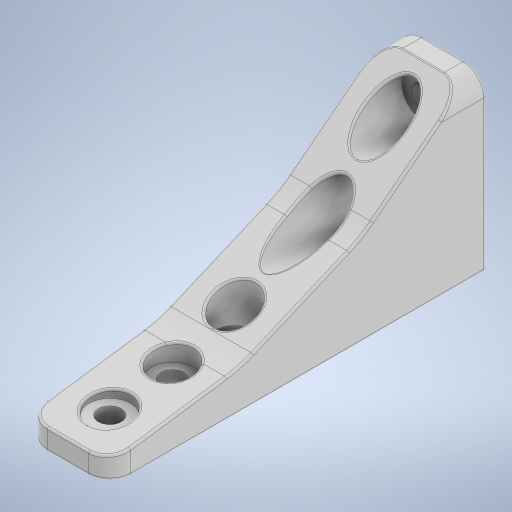
# Autodesk Inventor part: BraketBack
Saved by Autodesk Inventor 2024 (Build 280153000, 153)
## iProperties
Created: 2023-12-26
Part Number: BraketBack
Material: Generisch
Document SubType Name: Modeling
Designer: denni
Density: 1 g/cm^3
Appearance: Vorgabe
Author: denni
Autodesk Inventor part; units mm, degrees
ref_plane "YZ Plane" through (0, 0, 0) normal (1, 0, 0) x (0, 1, 0)
ref_plane "XZ Plane" through (0, 0, 0) normal (0, 1, 0) x (-1, 0, 0)
ref_plane "XY Plane" through (0, 0, 0) normal (0, 0, 1) x (1, 0, 0)
sketch "Skizze1" plane through (0, 0, 0) normal (1, 0, 0) x (0, 1, 0)
  line L0 (0, 90) -> (0, 0)
  line L1 (0, 0) -> (41, 0)
  line L2 (41, 0) -> (41, 5)
  line L3 (0, 90) -> (5, 90)
  line L4 (5, 90) -> (9.3569, 58.8179)
  line L5 (9.3569, 58.8179) -> (21.6358, 29.826)
  line L6 (21.6358, 29.826) -> (41, 5)
  dimension "d0" = 90
  dimension "d1" = 41
  dimension "d2" = 5
  dimension "d3" = 165
  dimension "d4" = 165
  constraints: 14 end point, 3 equal length, 2 vertical, 1 horizontal, 1 perpendicular
  measures "d0" distance of L0.start L0.end
  measures "d1" distance of L0.end L1.end
  measures "d2" distance of L1.end L2.end
  measures "d3" angle of L5 L6
  measures "d4" angle of L4 L5
extrude "Extrusion1" add sketch "Skizze1" along normal blind 20
fillet "Rundung1" radius 25 2 edges at (10, 9.3569, 58.8179) (10, 21.6358, 29.826)
sketch "Skizze4" plane through (0, 41, 5) normal (0, 1, 0) x (1, 0, 0)
  line L0 (0, -85) -> (20, -85) construction
  line L1 (0, -57.0776) -> (0, -85) construction
  point P0 (0, 5)
  point P1 (10, -75)
  point P2 (10, -60)
  point P3 (10, -45)
  dimension "d10" = 10
  dimension "d11" = 15
  dimension "d12" = 15
  dimension "d13" = 10
  dimension "d14" = 10
  dimension "d15" = 10
  measures "d10" distance from line of L0 point (10, -75)
  measures "d11" distance of point (10, -60) point (10, -75)
  measures "d12" distance of point (10, -45) point (10, -60)
  measures "d13" distance from line of L1 point (10, -75)
  measures "d14" distance from line of L1 point (10, -60)
  measures "d15" distance from line of L1 point (10, -45)
hole "Bohrung1" at (10, 41, 80) at (10, 41, 65) at (10, 41, 50) direction (0, -1, 0) diameter 5.5 end through all counterbore diameter 10 counterbore depth 36 clearance for "Inbusschraube ISO 4762" size "M5" standard "ISO"
sketch "Skizze6" plane through (0, 0, 90) normal (0, 0, 1) x (1, 0, 0)
  line L0 (20, 41) -> (20, 23.6601) projected
  line L1 (0, 41) -> (20, 41) projected
  point P0 (0, 0)
  point P1 (10, 33.5)
  point P2 (10, 21)
  dimension "d23" = 10
  dimension "d24" = 10
  dimension "d25" = 7.5
  dimension "d26" = 12.5
  measures "d23" distance from line of L0 point (10, 33.5)
  measures "d24" distance from line of L0 point (10, 21)
  measures "d25" distance from line of L1 point (10, 33.5)
  measures "d26" distance of point (10, 33.5) point (10, 21)
hole "Bohrung2" at (10, 33.5, 90) at (10, 21, 90) direction (0, 0, -1) diameter 5.5 end through all counterbore diameter 10 counterbore depth 85 clearance for "Inbusschraube ISO 4762" size "M5" standard "ISO"
fillet "Rundung2" radius 5 4 edges at (0, 2.5, 90) (20, 2.5, 90) (0, 41, 2.5) (20, 41, 2.5)
fillet "Rundung3" radius 0.5 38 edges at (20, 9.5648, 58.8754) (20, 7.3, 73.5388) (18.5355, 5.2046, 88.5355) (10, 5, 90) (1.4645, 5.2046, 88.5355) (0, 7.3, 73.5388) (0, 9.5648, 58.8754) (0, 15.4963, 44.322) (0, 21.8218, 29.9354) (0, 29.83, 19.3205) (1.4645, 39.5355, 6.8775) (10, 41, 5) (18.5355, 39.5355, 6.8775) (20, 29.83, 19.3205) (20, 21.8218, 29.9354) (20, 15.4963, 44.322) (18.5355, 39.5355, 0) (10, 41, 0) (1.4645, 39.5355, 0) (0, 18, 0) (20, 18, 0) (18.5355, 0, 88.5355) (10, 0, 90) (1.4645, 0, 88.5355) (0, 0, 42.5) (20, 0, 42.5) (10, 0, 0) (5.5496, 8.1747, 67.279) (14.4504, 8.1747, 67.279) (10, 7.0959, 75) (10, 9.2818, 60) (10, 15.2092, 45) (5.068, 21.8216, 29.9357) (14.9322, 21.8208, 29.9371) (10, 26, 24.2309) (13.2986, 17.2424, 40.1993) (6.7014, 17.2424, 40.1993) (10, 38.5, 8.2051)
